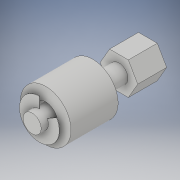
# Autodesk Inventor part: Float_Switch
Saved by Autodesk Inventor 2018 (Build 220112000, 112)
## iProperties
Created: 2019-07-25
Part Number: Float_Switch
Material: Generic
Document SubType Name: Modeling
Designer: micha
Density: 1 g/cm^3
Appearance: Default
Author: micha
Autodesk Inventor part; units mm, degrees
ref_plane "YZ Plane" through (0, 0, 0) normal (1, 0, 0) x (0, 1, 0)
ref_plane "XZ Plane" through (0, 0, 0) normal (0, 1, 0) x (-1, 0, 0)
ref_plane "XY Plane" through (0, 0, 0) normal (0, 0, 1) x (1, 0, 0)
sketch "Sketch1" plane through (0, 0, 0) normal (0, 0, 1) x (1, 0, 0)
  circle A0 centre (0, 0) radius 3.9688
  dimension "d0" = 7.9375
  constraints: 1 centre point, 1 coincident
  measures "d0" diameter of A0
extrude "Extrusion1" add sketch "Sketch1" along normal blind 50.8
ref_plane "Work Plane1" through (0, 0, 47.625) normal (0, 0, 1) x (1, 0, 0)
sketch "Sketch2" plane through (0, 0, 47.625) normal (0, 0, 1) x (1, 0, 0)
  arc A0 (0, 8.7313) -> (7.5615, 4.3656) centre (0, 0) ccw
  line L0 (0, 0) -> (0, 8.7313)
  line L1 (0, 0) -> (7.5615, 4.3656)
  dimension "d4" = 17.4625
  dimension "d5" = 60
  constraints: 4 end point, 2 point on circle, 1 centre point, 1 coincident
  measures "d4" diameter of A0
  measures "d5" angle of L1 L0
extrude "Extrusion2" add sketch "Sketch2" against normal blind 0.254
ref_plane "Work Plane2" through (0, 0, 44.831) normal (0, 0, -1) x (-1, 0, 0)
sketch "Sketch3" plane through (0, 0, 44.831) normal (0, 0, -1) x (-1, 0, 0)
  circle A0 centre (0, 0) radius 3.9687 projected
  circle A1 centre (0, 0) radius 11.1125
  circle A2 centre (0, 0) radius 5.2387
  dimension "d9" = 22.225
  dimension "d10" = 1.27
  constraints: 2 centre point, 1 coincident
  measures "d9" diameter of A1
  measures "d10" radial gap between concentric circles of A0 A2
extrude "Extrusion3" add sketch "Sketch3" along normal blind 20.6375 contours A1
sketch "Sketch4" plane through (0, 0, 0) normal (0, 0, -1) x (-1, 0, 0)
  circle A0 centre (0, 0) radius 3.9687 projected
  line L0 (8.2489, 0) -> (4.1244, -7.1437)
  line L1 (4.1244, -7.1437) -> (-4.1244, -7.1437)
  line L2 (-4.1244, -7.1437) -> (-8.2489, 0)
  line L3 (-8.2489, 0) -> (-4.1244, 7.1438)
  line L4 (-4.1244, 7.1438) -> (4.1244, 7.1438)
  line L5 (4.1244, 7.1438) -> (8.2489, 0)
  dimension "d13" = 14.2875
  constraints: 12 end point, 1 coincident, 1 horizontal, 13 other
  measures "d13" distance between parallel lines of L1 L4
extrude "Extrusion4" add sketch "Sketch4" against normal blind 12.7
body "Solid1"
